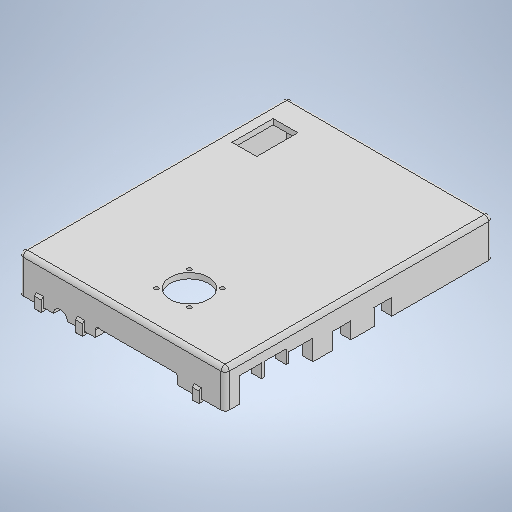
# Autodesk Inventor part: Electronic Lid - Final
Saved by Autodesk Inventor 2025.2 (Build 292293000, 293)
## iProperties
Created: 2025-03-21
Part Number: Electronic Lid - Final
Material: Generic
Document SubType Name: Modeling
Designer: caomi
Density: 1 g/cm^3
Appearance: Default
Author: caomi
Autodesk Inventor part; units mm, degrees
ref_plane "YZ Plane" through (0, 0, 0) normal (1, 0, 0) x (0, 1, 0)
ref_plane "XZ Plane" through (0, 0, 0) normal (0, 1, 0) x (-1, 0, 0)
ref_plane "XY Plane" through (0, 0, 0) normal (0, 0, 1) x (1, 0, 0)
sketch "Sketch1" plane through (0, 0, 0) normal (0, 1, 0) x (-1, 0, 0)
  line L0 (0, 0) -> (-135, 0)
  line L1 (-135, 0) -> (-135, 180)
  line L2 (-135, 180) -> (0, 180)
  line L3 (0, 180) -> (0, 0)
  dimension "d9" = 135
  dimension "d21" = 180
  constraints: 8 end point, 2 parallel, 1 horizontal, 1 perpendicular
  measures "d9" distance of L1.end L2.end
  measures "d21" distance of L2.end L0.start
extrude "Extrusion1" add sketch "Sketch1" along normal blind 20
shell "Shell1" thickness 7.5 outward yes removed faces 1 at (90, 0, 60)
sketch "Sketch2" plane through (0, 0, 0) normal (0, -1, 0) x (1, 0, 0)
  line L0 (142.5, 187.5) -> (142.5, -7.5) projected
  line L1 (142.5, 177) -> (135, 177)
  line L2 (135, 177) -> (135, 161)
  line L3 (135, 161) -> (142.5, 161)
  line L4 (142.5, 161) -> (142.5, 177)
  line L5 (142.5, 159) -> (135, 159)
  line L6 (135, 159) -> (135, 143)
  line L7 (135, 143) -> (142.5, 143)
  line L8 (142.5, 143) -> (142.5, 159)
  line L9 (0, 180) -> (135, 180) projected
  line L10 (142.5, 141) -> (135, 141)
  line L11 (135, 141) -> (135, 123.5)
  line L12 (135, 123.5) -> (142.5, 123.5)
  line L13 (142.5, 123.5) -> (142.5, 141)
  line L14 (135, 180) -> (135, 0) projected
  line L15 (142.5, 109.5) -> (135, 109.5)
  line L16 (135, 109.5) -> (135, 95.86)
  line L17 (135, 95.86) -> (142.5, 95.86)
  line L18 (142.5, 95.86) -> (142.5, 109.5)
  line L19 (142.5, 79) -> (135, 79)
  line L20 (135, 79) -> (135, 66)
  line L21 (135, 66) -> (142.5, 66)
  line L22 (142.5, 66) -> (142.5, 79)
  line L23 (-7.5, 187.5) -> (142.5, 187.5) projected
  line L24 (108, 187.5) -> (48, 187.5)
  line L25 (48, 187.5) -> (48, 180)
  line L26 (48, 180) -> (108, 180)
  line L27 (108, 180) -> (108, 187.5)
  point P0 (138.75, 161)
  point P1 (142.5, 66)
  point P2 (135, 79)
  point P3 (142.5, 95.86)
  point P4 (135, 109.5)
  point P5 (142.5, 123.5)
  point P6 (142.5, 161)
  point P7 (108, 180)
  point P8 (48, 187.5)
  dimension "d10" = 3
  dimension "d12" = 21
  dimension "d16" = 70.5
  dimension "d18" = 101
  dimension "d19" = 13
  dimension "d20" = 13.64
  dimension "d22" = 27
  dimension "d23" = 87
  dimension "d27" = 19
  dimension "d28" = 37
  dimension "d29" = 39
  dimension "d30" = 56.5
  constraints: 48 end point, 12 parallel, 12 point on line, 6 horizontal, 6 perpendicular, 1 midpoint
  measures "d10" distance between parallel lines of L1 L9
  measures "d12" distance from line of L5 L9.end
  measures "d16" distance of L9.end L15.end
  measures "d18" distance from line of L9.end L19
  measures "d19" distance of L21.end L19.start
  measures "d20" distance of L17.end L15.start
  measures "d22" distance of L9.end L26.end
  measures "d23" distance of L9.end L25.end
  measures "d27" distance from line of L9.end L3
  measures "d28" vertical distance of L9.end L7.end
  measures "d29" vertical distance of L9.end L10.start
  measures "d30" vertical distance of L9.end L12.end
extrude "Board Ports" cut sketch "Sketch2" against normal blind 18 contours L0 L3 L2 L1 | L0 L7 L6 L5
extrude "Extrusion9" cut sketch "Sketch2" against normal blind 7 contours L27 L9 L25 L23
fillet "Fillet4" radius 2 2 edges at (48, 7, 183.75) (108, 7, 183.75)
extrude "Extrusion10" cut sketch "Sketch2" against normal blind 8 contours L0 L5 L14 L3 | L0 L10 L14 L7
extrude "Extrusion11" cut sketch "Sketch2" against normal blind 15 contours L0 L12 L11 L10
extrude "Extrusion12" cut sketch "Sketch2" against normal blind 12 contours L0 L17 L14 L15 | L0 L21 L14 L19
fillet "Fillet1" radius 3 8 edges at (142.5, 13.75, 187.5) (-7.5, 13.75, 187.5) (142.5, 13.75, -7.5) (-7.5, 13.75, -7.5) (-7.5, 27.5, 90) (67.5, 27.5, -7.5) (67.5, 27.5, 187.5) (142.5, 27.5, 90)
ref_plane "Work Plane6" through (122.5, 0, 177) normal (1, 0, 0) x (0, 0, -1)
ref_plane "Work Plane7" through (37.5, 0, 177) normal (1, 0, 0) x (0, 0, -1)
ref_plane "Work Plane8" through (12.5, 0, 177) normal (1, 0, 0) x (0, 0, -1)
ref_plane "Work Plane9" through (7.5, 0, 177) normal (1, 0, 0) x (0, 0, -1)
sketch "Sketch3" plane through (142.5, 0, 95.86) normal (1, 0, 0) x (0, 0, -1)
  line L0 (-91.64, 24.5) -> (-91.64, 0) projected
  line L1 (-91.64, 0) -> (-90.44, 0)
  line L2 (-90.44, 0) -> (-90.44, -2.5)
  line L3 (-90.44, -2.5) -> (-91.64, -2.5)
  line L4 (-91.64, -2.5) -> (-91.64, 0)
  line L5 (-90.44, -2.5) -> (-89.44, -1.5)
  line L6 (-89.44, -1.5) -> (-90.44, -0.5)
  line L7 (-89.44, -1.5) -> (-90.44, -1.5) construction
  line L8 (-88.64, 24.5) -> (100.36, 24.5) projected
  line L9 (5.86, 51.3756) -> (5.86, -39.6704) construction
  line L10 (103.36, 0) -> (102.16, 0)
  line L11 (102.16, 0) -> (102.16, -2.5)
  line L12 (102.16, -2.5) -> (103.36, -2.5)
  line L13 (103.36, -2.5) -> (103.36, 0)
  line L14 (102.16, -2.5) -> (101.16, -1.5)
  line L15 (101.16, -1.5) -> (102.16, -0.5)
  line L16 (101.16, -1.5) -> (102.16, -1.5) construction
  line L17 (-91.64, -2.5) -> (-93.14, -2.5)
  line L18 (-93.14, -2.5) -> (-93.14, 5.5)
  line L19 (-93.14, 5.5) -> (-91.64, 5.5)
  line L20 (-91.64, 5.5) -> (-91.64, -2.5)
  line L21 (-93.14, 5.5) -> (-91.64, 7)
  circle A0 centre (-92.39, -2.5) radius 0.4
  line L22 (104.86, -2.5) -> (104.86, 5.5)
  line L23 (104.86, 5.5) -> (103.36, 5.5)
  line L24 (104.86, 5.5) -> (103.36, 7)
  circle A1 centre (104.11, -2.5) radius 0.4
  line L25 (103.36, -2.5) -> (104.86, -2.5)
  line L26 (103.36, 0) -> (103.36, 24.5) projected
  line L27 (103.36, 0) -> (100.36, 0) projected
  point P0 (95.86, 0)
  point P1 (5.86, 24.5)
  point P2 (-92.79, -2.5)
  point P3 (-91.99, -2.5)
  point P4 (103.71, -2.5)
  point P5 (104.51, -2.5)
  dimension "d35" = 1.2
  dimension "d36" = 2.5
  dimension "d37" = 1
  dimension "d38" = 45
  dimension "d128" = 45
  dimension "d129" = 1.5
  dimension "d130" = 0.8
  dimension "d133" = 8
  constraints: 48 end point, 12 symmetric about line, 6 point on line, 4 parallel, 3 perpendicular, 2 centre point, 2 horizontal, 2 midpoint, 1 vertical, 2 other
  measures "d35" distance of L2.end L3.end
  measures "d36" distance of L3.end L0.end
  measures "d37" distance of L5.end L7.end
  measures "d38" angle of L2 L5
  measures "d128" angle of L21 L19
  measures "d129" distance between parallel lines of L20 L18
  measures "d130" diameter of A0
  measures "d133" distance from line of L17.end L19
extrude "Extrusion3" add sketch "Sketch3" along normal mid plane 5 from surface at -20 contours L0 L19 L21 | L0 L4 L17 A0 L18 L19 | L1 L2 L3 L4 | A0 L17 | L6 L5 L2 picked at (-92.3739, -2.3676)
extrude "Extrusion25" cut sketch "Sketch3" along normal mid plane 4 from surface at -20 contours A0 L17 picked at (-92.3739, -2.3676)
extrude "Extrusion8" add sketch "Sketch3" along normal mid plane 5 from surface at -105 contours L0 L19 L21 | L0 L4 L17 A0 L18 L19 | L1 L2 L3 L4 | A0 L17 | L6 L5 L2 picked at (-92.3739, -2.3676)
extrude "Extrusion26" cut sketch "Sketch3" along normal mid plane 4 from surface at -105 contours A0 L17 picked at (-92.3739, -2.3676)
extrude "Extrusion5" add sketch "Sketch3" along normal mid plane 5 from surface at -135 contours L0 L19 L21 | L0 L4 L17 A0 L18 L19 | L1 L2 L3 L4 | A0 L17 | L6 L5 L2 picked at (-92.3739, -2.3676)
extrude "Extrusion27" cut sketch "Sketch3" along normal mid plane 4 from surface at -135 contours A0 L17 picked at (-92.3739, -2.3676)
extrude "Extrusion6" add sketch "Sketch3" along normal mid plane 5 from surface at -20 contours L13 L12 L11 L10 | L26 L23 L22 L25 A1 L13 | L26 L24 L23 | L11 L14 L15 | A1 L25 picked at (104.1261, -2.3676)
extrude "Extrusion28" cut sketch "Sketch3" along normal mid plane 4 from surface at -20 contours A1 L25 picked at (104.1261, -2.3676)
extrude "Extrusion7" add sketch "Sketch3" along normal mid plane 5 from surface at -130 contours L13 L12 L11 L10 | L26 L23 L22 L25 A1 L13 | L26 L24 L23 | L11 L14 L15 | A1 L25 picked at (104.1261, -2.3676)
extrude "Extrusion29" cut sketch "Sketch3" along normal mid plane 4 from surface at -130 contours A1 L25 picked at (104.1261, -2.3676)
sketch "Sketch4" plane through (48, 7, 187.5) normal (0, 0, 1) x (1, 0, 0)
  line L0 (-38, -7) -> (-13, -7) projected
  circle A0 centre (-25.5, -7) radius 5
  line L1 (-55.5, 17.5) -> (-55.5, -7) projected
  point P0 (-48, -7)
  dimension "d64" = 30
  dimension "d67" = 10
  constraints: 1 centre point, 1 midpoint
  measures "d64" distance from line of L1 A0.centre
  measures "d67" diameter of A0
extrude "DC opening" cut sketch "Sketch4" against normal up to surface (7.5 mm away)
ref_plane "Work Plane10" through (0, -7, 180) normal (0, -1, 0) x (1, 0, 0)
sketch "Sketch5" plane through (0, 0, 180) normal (0, -1, 0) x (1, 0, 0)
  line L0 (27.75, 1.5) -> (17.25, 1.5)
  line L1 (17.25, 1.5) -> (15.5, -11.5)
  line L2 (15.5, -11.5) -> (29.5, -11.5)
  line L3 (29.5, -11.5) -> (27.75, 1.5)
  line L4 (22.5, 3.5405) -> (22.5, -12.0447) construction
  line L5 (17.5, 7.5) -> (27.5, 7.5) projected
  line L6 (-7.5, -184.5) -> (-7.5, 4.5) projected
  line L7 (17.5, 0) -> (17.5, 7.5) projected
  line L8 (10, 7.5) -> (17.5, 7.5) projected
  line L9 (10, 7.5) -> (10, 6.3) projected
  line L10 (10, 6.3) -> (5, 6.3) projected
  line L11 (5, 7.5) -> (5, 6.3) projected
  line L12 (-4.5, 7.5) -> (5, 7.5) projected
  arc A0 (-4.5, 7.5) -> (-7.5, 4.5) centre (-4.5, 4.5) ccw projected
  arc A1 (-7.5, -184.5) -> (-4.5, -187.5) centre (-4.5, -184.5) ccw projected
  line L13 (10, -187.5) -> (-4.5, -187.5) projected
  line L14 (10, -186.3) -> (10, -187.5) projected
  line L15 (10, -186.3) -> (15, -186.3) projected
  line L16 (15, -186.3) -> (15, -187.5) projected
  line L17 (120, -187.5) -> (15, -187.5) projected
  line L18 (120, -186.3) -> (120, -187.5) projected
  line L19 (120, -186.3) -> (125, -186.3) projected
  line L20 (125, -186.3) -> (125, -187.5) projected
  line L21 (139.5, -187.5) -> (125, -187.5) projected
  arc A2 (139.5, -187.5) -> (142.5, -184.5) centre (139.5, -184.5) ccw projected
  line L22 (142.5, -114) -> (142.5, -184.5) projected
  line L23 (142.5, -114) -> (135, -114) projected
  line L24 (135, -114) -> (135, -180) projected
  line L25 (135, -180) -> (0, -180) projected
  line L26 (0, -180) -> (0, 0) projected
  line L27 (0, 0) -> (17.5, 0) projected
  dimension "d69" = 10.5
  dimension "d70" = 14
  dimension "d71" = 13
  dimension "d72" = 6
  dimension "d73" = 30
  constraints: 10 end point, 2 horizontal, 1 vertical, 1 other
  measures "d69" distance of L0.start L0.end
  measures "d70" distance of L1.end L2.end
  measures "d71" distance between parallel lines of L2 L0
  measures "d72" distance between parallel lines of L5 L0
  measures "d73" distance between parallel lines of L6 L4
extrude "Extrusion14" cut sketch "Sketch5" against normal blind 3 contours L3 L2 L1 L27 L7 L0 | L7 L27 L1 L0
sketch "Sketch9" plane through (0, 0, 0) normal (0, -1, 0) x (1, 0, 0)
  line L0 (0, 0) -> (0, 180) projected
  line L1 (-7.5, -4.5) -> (-7.5, 184.5) projected
  line L2 (0, 114.55) -> (-7.5, 114.55)
  line L3 (-7.5, 114.55) -> (-7.5, 101.35)
  line L4 (-7.5, 101.35) -> (0, 101.35)
  line L5 (0, 101.35) -> (0, 114.55)
  line L6 (0, 115) -> (-6.2, 115)
  line L7 (-6.2, 115) -> (-6.2, 100.9)
  line L8 (-6.2, 100.9) -> (0, 100.9)
  line L9 (0, 100.9) -> (0, 115)
  line L10 (4.3299, 107.95) -> (-13.6963, 107.95) construction
  line L11 (0, 116.95) -> (5, 116.95)
  line L12 (5, 116.95) -> (5, 98.95)
  line L13 (5, 98.95) -> (0, 98.95)
  line L14 (0, 98.95) -> (0, 116.95)
  line L15 (0, 114.55) -> (5, 114.55)
  line L16 (5, 114.55) -> (5, 101.35)
  line L17 (5, 101.35) -> (0, 101.35)
  line L18 (0, 101.35) -> (0, 114.55)
  point P0 (0, 107.95)
  point P1 (-6.2, 114.55)
  point P2 (-7.5, 114.55)
  point P3 (-6.2, 101.35)
  point P4 (0, 100.9)
  point P5 (0, 101.35)
  point P6 (0, 98.95)
  dimension "d104" = 13.2
  dimension "d105" = 14.1
  dimension "d107" = 6.2
  dimension "d108" = 18
  dimension "d109" = 5
  dimension "d117" = 115
  constraints: 34 end point, 8 parallel, 6 point on line, 5 horizontal, 4 perpendicular, 1 midpoint, 2 other
  measures "d104" distance between parallel lines of L4 L2
  measures "d105" distance of L6.end L7.end
  measures "d107" distance of L6.start L6.end
  measures "d108" distance of L11.end L12.end
  measures "d109" distance between parallel lines of L5 L12
  measures "d117" vertical distance of L0.start L6.end
extrude "DC Motor JST-PH slot" cut sketch "Sketch9" against normal blind 1.7 contours L8 L7 L4 L0 | L4 L7 L2 L0 | L2 L7 L6 L0 | L4 L1 L2 L7
extrude "JST-PH slot reinforce" add sketch "Sketch9" against normal up to surface (20 mm away) contours L0 L17 L12 L13 | L0 L11 L12 L15
sketch "Sketch11" plane through (5, 0, 98.95) normal (0, 0, -1) x (-1, 0, 0)
  line L0 (0, 20) -> (5, 20) projected
  line L1 (0, 0) -> (0, 20) projected
  line L2 (5, 20) -> (5, 0) projected
  line L3 (0, 3) -> (5, 8)
  dimension "d121" = 45
  dimension "d122" = 8
  constraints: 2 end point, 2 point on line
  measures "d121" angle of L2 L3
  measures "d122" distance of L2.end L3.end
extrude "Material reduction" cut sketch "Sketch11" against normal up to surface (18 mm away)
pattern_linear "Rectangular Pattern1" count 4 spacing 16 along (0, 0, -1) of "DC Motor JST-PH slot", "JST-PH slot reinforce", "Material reduction"
fillet "Fillet2" radius 1 5 edges at (122.5, -1.5, 185.3) (37.5, -1.5, 185.3) (7.5, -1.5, 185.3) (122.5, -1.5, -5.3) (12.5, -1.5, -5.3)
fillet "Fillet3" radius 1 10 edges at (125, 0, -6.9) (120, 0, -6.9) (15, 0, -6.9) (10, 0, -6.9) (5, 0, 186.9) (10, 0, 186.9) (35, 0, 186.9) (40, 0, 186.9) (120, 0, 186.9) (125, 0, 186.9)
sketch "Sketch7" plane through (0, 20, 180) normal (0, -1, 0) x (1, 0, 0)
  line L0 (2, -168) -> (20, -168)
  line L1 (20, -168) -> (20, -138)
  line L2 (20, -138) -> (2, -138)
  line L3 (2, -138) -> (2, -168)
  line L4 (135, -180) -> (0, -180) projected
  line L5 (0, -180) -> (0, 0) projected
  line L6 (63.3636, -45.6128) -> (93.8636, -45.6128)
  line L7 (93.8636, -45.6128) -> (93.8636, -15.1128)
  line L8 (93.8636, -15.1128) -> (63.3636, -15.1128)
  line L9 (63.3636, -15.1128) -> (63.3636, -45.6128)
  line L10 (48.5433, -30.3628) -> (101.3697, -30.3628) construction
  line L11 (78.6136, -33.9742) -> (78.6136, -85.2203) construction
  circle A0 centre (66.6136, -42.3628) radius 1.5
  circle A1 centre (66.6136, -18.3628) radius 1.5
  circle A2 centre (90.6136, -42.3628) radius 1.5
  circle A3 centre (90.6136, -18.3628) radius 1.5
  circle A4 centre (78.6136, -30.3628) radius 14
  point P0 (0, -95.4083)
  dimension "d83" = 12
  dimension "d84" = 42
  dimension "d85" = 2
  dimension "d86" = 20
  dimension "d91" = 30.5
  dimension "d92" = 30.5
  dimension "d93" = 3
  dimension "d95" = 24
  dimension "d96" = 24
  dimension "d101" = 28
  constraints: 20 end point, 5 centre point, 4 parallel, 3 horizontal, 3 symmetric about line, 2 perpendicular, 2 point on line, 1 vertical, 5 other
  measures "d83" distance between parallel lines of L4 L0
  measures "d84" distance from line of L4 L2.end
  measures "d85" distance between parallel lines of L5 L3
  measures "d86" distance between parallel lines of L5 L1
  measures "d91" distance of L6.end L7.end
  measures "d92" distance of L6.start L6.end
  measures "d93" diameter of A0
  measures "d95" distance of A3.centre A2.centre
  measures "d96" distance of A2.centre A0.centre
  measures "d101" diameter of A4
extrude "Motor driver heat sink hole" cut sketch "Sketch7" against normal blind 20 contours L3 L2 L1 L0
extrude "Fan recess face" cut sketch "Sketch7" against normal blind 2 contours L9 L8 L7 L6 | A0 | A1 | A2 | A3 | A4
extrude "Fan mounting holes" cut sketch "Sketch7" against normal through all contours A0 | A1 | A2 | A3
extrude "Fan opening" cut sketch "Sketch7" against normal blind 10 contours A4
sketch "Sketch8" plane through (0, 20, 180) normal (0, -1, 0) x (1, 0, 0)
  line L0 (2, -138) -> (20, -138) projected
  line L1 (20, -138) -> (20, -168) projected
  line L2 (20, -168) -> (2, -168) projected
  line L3 (2, -168) -> (2, -138) projected
  line L4 (0, 0) -> (135, 0) projected
  line L5 (0, -180) -> (0, 0) projected
  line L6 (0, -92.3585) -> (0, -87.6415) projected
  line L7 (0, -180) -> (0, 0) projected
  line L8 (135, -180) -> (0, -180) projected
  line L9 (135, 0) -> (135, -180) projected
extrude "Extrusion17" cut sketch "Sketch8" against normal blind 3.5
sketch "Sketch10" plane through (-7.5, 0, 184.5) normal (-1, 0, 0) x (0, 0, 1)
  line L0 (-101.95, 0) -> (-99.15, 0) projected
  line L1 (-69.95, 0) -> (0, 0) projected
  line L2 (-75.55, 15) -> (-125.55, 15) construction
  line L3 (-75.55, 20) -> (-125.55, 20)
  line L4 (-125.55, 10) -> (-75.55, 10)
  arc A0 (-75.55, 10) -> (-75.55, 20) centre (-75.55, 15) ccw
  arc A1 (-125.55, 20) -> (-125.55, 10) centre (-125.55, 15) ccw
  point P0 (-184.5, 0)
  point P1 (-100.55, 15)
  point P2 (-100.55, 0)
  dimension "d118" = 50
  dimension "d119" = 5
  dimension "d120" = 15
  constraints: 8 end point, 4 point on circle, 4 tangent, 2 centre point, 2 midpoint, 1 horizontal, 1 parallel, 1 vertical alignment
  measures "d118" distance of L2.start L2.end
  measures "d119" radius of A1
  measures "d120" distance between parallel lines of L1 L2
extrude "Extra cable slot" cut sketch "Sketch10" against normal blind 10
equation "\"d92\" = d91"
equation "\"d96\" = d95"
body "Solid1"
